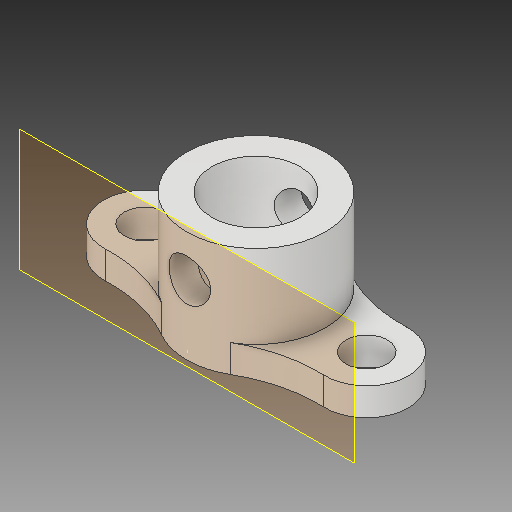
# Autodesk Inventor part: EncoderWheelAdapter
Saved by Autodesk Inventor 2018 (Build 220112000, 112)
## iProperties
Created: 2018-03-25
Part Number: EncoderWheelAdapter
Material: ABS Plastic
Document SubType Name: Modeling
Designer: mansu
Density: 1.06 g/cm^3
Appearance: Smooth - White
Mass: 0.492256 g
Surface Area: 7.06553 cm^2
Volume: 0.464392 cm^3
Author: mansu
Autodesk Inventor part; units mm, degrees
ref_plane "YZ Plane" through (0, 0, 0) normal (1, 0, 0) x (0, 1, 0)
ref_plane "XZ Plane" through (0, 0, 0) normal (0, 1, 0) x (-1, 0, 0)
sketch "Sketch1" plane through (0, 0, 0) normal (0, 1, 0) x (-1, 0, 0)
  circle A0 centre (0, 0) radius 3.175
  arc A1 (2.5, 4.3301) -> (2.5, -4.3301) centre (0, 0) ccw
  circle A2 centre (8, 0) radius 1.5
  circle A3 centre (-8, 0) radius 1.5
  arc A4 (-7.8846, 2.9978) -> (-7.8846, -2.9978) centre (-8, 0) ccw
  arc A5 (-2.5, -4.3301) -> (-7.8846, -2.9978) centre (-7.5, -12.9904) ccw
  arc A6 (-7.8846, 2.9978) -> (-2.5, 4.3301) centre (-7.5, 12.9904) ccw
  line L0 (0, 0) -> (0, -5) construction
  arc A7 (7.8846, -2.9978) -> (7.8846, 2.9978) centre (8, 0) ccw
  arc A8 (7.8846, -2.9978) -> (2.5, -4.3301) centre (7.5, -12.9904) ccw
  arc A9 (2.5, 4.3301) -> (7.8846, 2.9978) centre (7.5, 12.9904) ccw
  arc A10 (2.5, -4.3301) -> (2.5, 4.3301) centre (0, 0) ccw
  dimension "d0" = 6.35
  dimension "d1" = 10
  dimension "d2" = 3
  dimension "d3" = 3
  dimension "d4" = 8
  dimension "d5" = 8
  dimension "d6" = 3
  dimension "d14" = 10
  constraints: 19 point on circle, 11 centre point, 7 symmetric about line, 4 tangent, 2 coincident, 2 end point, 2 horizontal alignment, 1 concentric, 1 equal radius, 1 vertical, 3 other
  measures "d0" diameter of A0
  measures "d1" diameter of A1
  measures "d2" diameter of A2
  measures "d3" diameter of A3
  measures "d4" distance of point (0, 0) A3.centre
  measures "d5" distance of point (0, 0) A2.centre
  measures "d6" radius of A4
  measures "d14" radius of A6
extrude "Extrusion1" add sketch "Sketch1" against normal blind 2
extrude "Extrusion2" add sketch "Sketch1" along normal blind 6 contours A10 A1
sketch "Sketch2" plane through (0, 0, 0) normal (0, 0, 1) x (1, 0, 0)
  circle A0 centre (0, 3) radius 1.5
  line L0 (5, 6) -> (5, 0) projected
  point P0 (0, 0)
  point P1 (5, 3)
  dimension "d11" = 3
  constraints: 1 centre point, 1 horizontal alignment, 1 midpoint, 1 vertical alignment
  measures "d11" diameter of A0
extrude "Extrusion3" cut sketch "Sketch2" along normal through all both and the other way through all
ref_plane "Work Plane1" through (0, 0, 5) normal (0, 0, 1) x (1, 0, 0)
body "Solid1"
